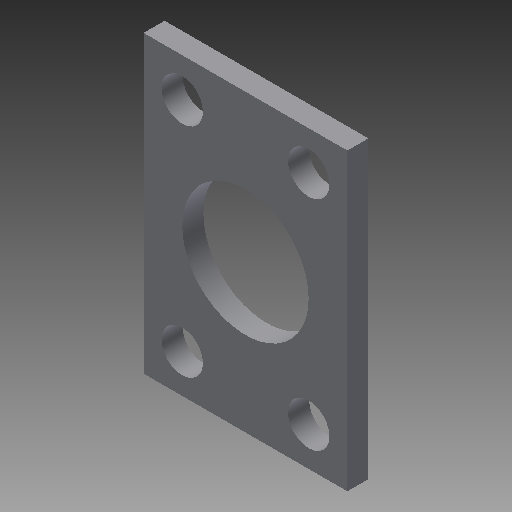
# Autodesk Inventor part: 零件7
Saved by Autodesk Inventor 2018 (Build 220112000, 112)
## iProperties
Created: 2017-07-24
Part Number: 零件7
Material: 一般
Document SubType Name: 板金
Designer: Alex
Density: 1 g/cm^3
Sheet Metal Rule: 預設
Appearance: 預設
Author: Alex
Autodesk Inventor part; units mm, degrees
ref_plane "YZ Plane" through (0, 0, 0) normal (1, 0, 0) x (0, 1, 0)
ref_plane "XZ Plane" through (0, 0, 0) normal (0, 1, 0) x (-1, 0, 0)
ref_plane "XY Plane" through (0, 0, 0) normal (0, 0, 1) x (1, 0, 0)
sketch "草圖1" plane through (0, 0, 0) normal (0, 0, 1) x (1, 0, 0)
  line L0 (-14.5, 21) -> (14.5, 21)
  line L1 (14.5, 21) -> (14.5, -21)
  line L2 (14.5, -21) -> (-14.5, -21)
  line L3 (-14.5, -21) -> (-14.5, 21)
  line L4 (-14.5, 21) -> (14.5, -21) construction
  line L5 (14.5, 21) -> (-14.5, -21) construction
  circle A0 centre (0, 0) radius 9
  line L6 (-9, 15.5) -> (9, 15.5) construction
  line L7 (9, 15.5) -> (9, -15.5) construction
  line L8 (9, -15.5) -> (-9, -15.5) construction
  line L9 (-9, -15.5) -> (-9, 15.5) construction
  line L10 (-9, 15.5) -> (9, -15.5) construction
  line L11 (9, 15.5) -> (-9, -15.5) construction
  circle A1 centre (-9, 15.5) radius 2.95
  circle A2 centre (9, 15.5) radius 2.95
  circle A3 centre (-9, -15.5) radius 2.95
  circle A4 centre (9, -15.5) radius 2.95
  dimension "d0" = 29
  dimension "d1" = 42
  dimension "d2" = 18
  dimension "d3" = 18
  dimension "d4" = 31
  dimension "d5" = 5.9
  dimension "d6" = 5.9
  dimension "d7" = 5.9
  dimension "d8" = 5.9
  constraints: 24 end point, 5 centre point, 5 coincident, 4 midpoint, 4 parallel, 2 horizontal, 2 perpendicular
  measures "d0" distance of L1.end L2.end
  measures "d1" distance of L0.end L1.end
  measures "d2" diameter of A0
  measures "d3" distance of L7.end L8.end
  measures "d4" distance of L6.end L7.end
  measures "d5" diameter of A1
  measures "d6" diameter of A2
  measures "d7" diameter of A3
  measures "d8" diameter of A4
extrude "擠出1" add sketch "草圖1" along normal blind 3
equation "\"折彎半徑\" = 厚度"
equation "\"折彎離隙寬度\" = 厚度"
equation "\"折彎離隙深度\" = 0.5 * 厚度"
equation "\"轉角離隙大小\" = 4 * 厚度"
equation "\"最小剩餘\" = 2 * 厚度"
equation "\"轉移半徑\" = 折彎半徑"
equation "\"Jacobi半徑大小\" = 折彎半徑"
equation "\"間隙大小\" = 厚度"
equation "\"厚度\" = 3.048"
